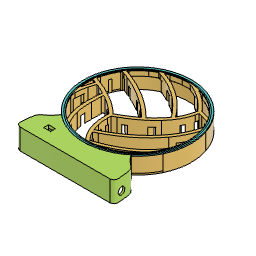
led_volleyball v4 (Autodesk Fusion 360 design; units mm, degrees)
Autodesk Fusion 360 part; units mm, degrees
(part 1 of 2)
sketch "Sketch1" plane through (0, 0, 0) normal (0, 0, 1) x (1, 0, 0) in component "volleyball"
  spline S0 degree 3 poles (6.9428, 90.0762) (-13.5515, 87.9678) (-33.2869, 78.5218) (-48.0462, 63.7625) knots 0 0 0 0 1 1 1 1
  spline S1 degree 3 poles (-48.0462, 63.7625) (-69.5526, 42.2982) (-78.872, 11.9784) (-73.137, -17.8354) knots 0 0 0 0 1 1 1 1
  spline S2 degree 3 poles (-73.137, -17.8354) (-69.7213, -35.5888) (-61.0344, -51.9084) (-48.0883, -64.8544) knots 0 0 0 0 1 1 1 1
  spline S3 degree 3 poles (-48.0883, -64.8544) (-27.594, -85.3066) (1.5451, -94.9212) (29.9252, -90.5778) knots 0 0 0 0 1 1 1 1
  spline S4 degree 3 poles (29.9252, -90.5778) (59.4438, -86.0656) (85.2093, -66.9629) (98.2397, -39.9744) knots 0 0 0 0 1 1 1 1
  spline S5 degree 3 poles (98.2397, -39.9744) (108.5291, -18.6788) (110.0472, 5.1048) (102.6253, 27.8341) knots 0 0 0 0 1 1 1 1
  spline S6 degree 3 poles (102.6253, 27.8341) (90.354, 65.4493) (54.8473, 90.9196) (15.4189, 90.4979) knots 0 0 0 0 1 1 1 1
  spline S7 degree 3 poles (15.4189, 90.4979) (12.72, 90.4558) (8.9248, 90.2449) (6.9428, 90.0762) knots 0 0 0 0 1 1 1 1
  spline S8 degree 3 poles (20.3105, 84.1725) (28.8709, 81.4737) (39.6242, 75.4434) (48.058, 68.612) knots 0 0 0 0 1 1 1 1
  spline S9 degree 3 poles (48.058, 68.612) (52.0641, 65.3649) (60.6667, 57.0997) (63.4921, 53.7683) knots 0 0 0 0 1 1 1 1
  line L0 (63.4921, 53.7683) -> (65.1789, 51.7864)
  line L1 (65.1789, 51.7864) -> (64.2933, 47.5694)
  spline S10 degree 3 poles (64.2933, 47.5694) (62.9017, 40.7801) (59.992, 33.3583) (55.9859, 26.5268) knots 0 0 0 0 1 1 1 1
  line L2 (55.9859, 26.5268) -> (54.9317, 24.7557)
  line L3 (54.9317, 24.7557) -> (52.781, 27.5811)
  spline S11 degree 3 poles (52.781, 27.5811) (45.57, 37.2379) (35.365, 47.5694) (24.9914, 55.666) knots 0 0 0 0 1 1 1 1
  spline S12 degree 3 poles (24.9914, 55.666) (13.2261, 64.8589) (-2.1236, 73.2928) (-14.7323, 77.4676) knots 0 0 0 0 1 1 1 1
  spline S13 degree 3 poles (-14.7323, 77.4676) (-18.1902, 78.6061) (-18.3167, 78.5218) (-10.6418, 81.052) knots 0 0 0 0 1 1 1 1
  spline S14 degree 3 poles (-10.6418, 81.052) (-4.2743, 83.1183) (-0.226, 84.046) (6.0994, 84.8472) knots 0 0 0 0 1 1 1 1
  spline S15 degree 3 poles (6.0994, 84.8472) (13.4369, 85.7328) (15.7141, 85.6484) (20.3105, 84.1725) knots 0 0 0 0 1 1 1 1
  spline S16 degree 3 poles (44.0519, 80.7568) (53.2027, 77.5941) (61.1728, 73.2928) (69.0163, 67.2626) knots 0 0 0 0 1 1 1 1
  spline S17 degree 3 poles (69.0163, 67.2626) (73.3597, 63.9312) (80.2334, 57.0997) (83.3961, 53.0936) knots 0 0 0 0 1 1 1 1
  line L4 (83.3961, 53.0936) -> (85.4202, 50.5213)
  line L5 (85.4202, 50.5213) -> (83.6069, 51.1538)
  spline S18 degree 3 poles (83.6069, 51.1538) (82.5948, 51.5333) (78.9683, 52.5454) (75.5104, 53.431) knots 0 0 0 0 1 1 1 1
  line L6 (75.5104, 53.431) -> (69.185, 55.0334)
  line L7 (69.185, 55.0334) -> (65.3475, 59.2925)
  spline S19 degree 3 poles (65.3475, 59.2925) (57.3353, 68.2325) (49.4496, 74.7265) (37.7265, 82.064) knots 0 0 0 0 1 1 1 1
  line L8 (37.7265, 82.064) -> (36.2506, 82.9918)
  line L9 (36.2506, 82.9918) -> (37.7265, 82.6966)
  spline S20 degree 3 poles (37.7265, 82.6966) (38.5277, 82.5701) (41.3953, 81.6845) (44.0519, 80.7568) knots 0 0 0 0 1 1 1 1
  spline S21 degree 3 poles (-20.4252, 74.094) (-7.0574, 70.1301) (10.6116, 60.5576) (23.5998, 50.2261) knots 0 0 0 0 1 1 1 1
  spline S22 degree 3 poles (23.5998, 50.2261) (29.7987, 45.3344) (43.3772, 31.6294) (47.9737, 25.6835) knots 0 0 0 0 1 1 1 1
  spline S23 degree 3 poles (47.9737, 25.6835) (49.9978, 23.0268) (51.6425, 20.6653) (51.6425, 20.3701) knots 0 0 0 0 1 1 1 1
  spline S24 degree 3 poles (51.6425, 20.3701) (51.6425, 18.852) (37.347, 3.3336) (32.5819, -0.2508) knots 0 0 0 0 1 1 1 1
  line L10 (32.5819, -0.2508) -> (31.0638, -1.4315)
  line L11 (31.0638, -1.4315) -> (26.889, 2.6168)
  spline S25 degree 3 poles (26.889, 2.6168) (16.3466, 12.9904) (0.9548, 24.5027) (-13.2985, 32.6414) knots 0 0 0 0 1 1 1 1
  spline S26 degree 3 poles (-13.2985, 32.6414) (-23.5035, 38.503) (-38.4315, 45.4188) (-49.0582, 49.214) knots 0 0 0 0 1 1 1 1
  line L12 (-49.0582, 49.214) -> (-52.9378, 50.6056)
  line L13 (-52.9378, 50.6056) -> (-51.3776, 52.5454)
  spline S27 degree 3 poles (-51.3776, 52.5454) (-46.4016, 58.7022) (-40.6243, 64.2685) (-34.3833, 68.9493) knots 0 0 0 0 1 1 1 1
  spline S28 degree 3 poles (-34.3833, 68.9493) (-30.9254, 71.5217) (-24.5578, 75.3169) (-24.0096, 75.1482) knots 0 0 0 0 1 1 1 1
  spline S29 degree 3 poles (-24.0096, 75.1482) (-23.7566, 75.0639) (-22.1119, 74.6) (-20.4252, 74.094) knots 0 0 0 0 1 1 1 1
  spline S30 degree 3 poles (75.7212, 48.202) (81.1611, 46.726) (86.6009, 44.7019) (89.2154, 43.226) knots 0 0 0 0 1 1 1 1
  spline S31 degree 3 poles (89.2154, 43.226) (90.354, 42.5934) (91.1974, 41.497) (92.5468, 39.009) knots 0 0 0 0 1 1 1 1
  line L14 (92.5468, 39.009) -> (94.318, 35.6776)
  line L15 (94.318, 35.6776) -> (92.7999, 29.8161)
  spline S32 degree 3 poles (92.7999, 29.8161) (85.0407, -0.6303) (61.1728, -29.432) (25.413, -51.4023) knots 0 0 0 0 1 1 1 1
  spline S33 degree 3 poles (25.413, -51.4023) (20.0997, -54.6494) (5.5512, -62.4929) (4.75, -62.5351) knots 0 0 0 0 1 1 1 1
  spline S34 degree 3 poles (4.75, -62.5351) (4.3705, -62.5351) (2.1355, -55.5771) (1.2499, -51.6975) knots 0 0 0 0 1 1 1 1
  spline S35 degree 3 poles (1.2499, -51.6975) (-0.0151, -46.0468) (-0.6477, -40.3118) (-0.6477, -34.4502) knots 0 0 0 0 1 1 1 1
  line L16 (-0.6477, -34.4502) -> (-0.6477, -28.4621)
  line L17 (-0.6477, -28.4621) -> (5.7621, -24.9621)
  spline S36 degree 3 poles (5.7621, -24.9621) (22.2925, -15.8956) (38.1061, -3.793) (48.2689, 7.5506) knots 0 0 0 0 1 1 1 1
  spline S37 degree 3 poles (48.2689, 7.5506) (59.1486, 19.6532) (65.7692, 31.3763) (68.7633, 43.9007) knots 0 0 0 0 1 1 1 1
  spline S38 degree 3 poles (68.7633, 43.9007) (69.3958, 46.473) (69.944, 48.8345) (70.0283, 49.1297) knots 0 0 0 0 1 1 1 1
  spline S39 degree 3 poles (70.0283, 49.1297) (70.197, 49.7622) (69.6488, 49.8466) (75.7212, 48.202) knots 0 0 0 0 1 1 1 1
  spline S40 degree 3 poles (-43.8292, 41.7079) (-24.7686, 34.0752) (-5.4128, 22.7738) (10.7381, 9.7856) knots 0 0 0 0 1 1 1 1
  spline S41 degree 3 poles (10.7381, 9.7856) (16.3466, 5.2734) (26.1299, -3.6243) (26.4673, -4.5099) knots 0 0 0 0 1 1 1 1
  spline S42 degree 3 poles (26.4673, -4.5099) (26.889, -5.6063) (12.5092, -15.3474) (2.3885, -20.8295) knots 0 0 0 0 1 1 1 1
  line L18 (2.3885, -20.8295) -> (-2.3345, -23.4018)
  line L19 (-2.3345, -23.4018) -> (-5.3285, -20.6186)
  spline S43 degree 3 poles (-5.3285, -20.6186) (-19.0757, -7.6304) (-41.3412, 5.2313) (-64.1971, 13.37) knots 0 0 0 0 1 1 1 1
  spline S44 degree 3 poles (-64.1971, 13.37) (-68.7514, 14.9724) (-68.6249, 14.7616) (-67.2754, 20.0749) knots 0 0 0 0 1 1 1 1
  spline S45 degree 3 poles (-67.2754, 20.0749) (-65.3356, 27.7919) (-60.7813, 38.6295) (-57.1969, 44.238) knots 0 0 0 0 1 1 1 1
  line L20 (-57.1969, 44.238) -> (-55.8897, 46.22)
  line L21 (-55.8897, 46.22) -> (-52.0101, 44.8284)
  spline S46 degree 3 poles (-52.0101, 44.8284) (-49.8595, 44.0272) (-46.1907, 42.6356) (-43.8292, 41.7079) knots 0 0 0 0 1 1 1 1
  spline S47 degree 3 poles (98.7879, 23.4906) (100.7699, 16.9544) (102.2458, 6.7494) (102.2458, -0.5459) knots 0 0 0 0 1 1 1 1
  spline S48 degree 3 poles (102.2458, -0.5459) (102.2458, -7.5039) (101.4868, -12.6064) (99.8843, -16.5282) knots 0 0 0 0 1 1 1 1
  spline S49 degree 3 poles (99.8843, -16.5282) (90.5649, -39.2154) (70.9139, -58.2338) (43.0399, -71.6015) knots 0 0 0 0 1 1 1 1
  spline S50 degree 3 poles (43.0399, -71.6015) (36.2506, -74.8907) (26.8046, -78.6016) (20.7322, -80.4571) knots 0 0 0 0 1 1 1 1
  line L22 (20.7322, -80.4571) -> (16.9792, -81.5957)
  line L23 (16.9792, -81.5957) -> (15.9249, -80.5836)
  spline S51 degree 3 poles (15.9249, -80.5836) (13.4369, -78.3064) (6.4368, -67.9328) (6.985, -67.4267) knots 0 0 0 0 1 1 1 1
  spline S52 degree 3 poles (6.985, -67.4267) (7.0693, -67.3424) (10.0212, -65.8243) (13.4791, -64.0953) knots 0 0 0 0 1 1 1 1
  spline S53 degree 3 poles (13.4791, -64.0953) (39.6663, -50.8541) (63.4499, -31.414) (78.7574, -10.7931) knots 0 0 0 0 1 1 1 1
  spline S54 degree 3 poles (78.7574, -10.7931) (86.5588, -0.2508) (93.0107, 12.3157) (96.4264, 23.575) knots 0 0 0 0 1 1 1 1
  spline S55 degree 3 poles (96.4264, 23.575) (96.9746, 25.3461) (97.5228, 26.6955) (97.6915, 26.5268) knots 0 0 0 0 1 1 1 1
  spline S56 degree 3 poles (97.6915, 26.5268) (97.818, 26.3582) (98.3241, 25.0087) (98.7879, 23.4906) knots 0 0 0 0 1 1 1 1
  spline S57 degree 3 poles (-66.0104, 8.5205) (-64.7453, 8.0988) (-63.6489, 7.7193) (-63.5645, 7.6771) knots 0 0 0 0 1 1 1 1
  spline S58 degree 3 poles (-63.5645, 7.6771) (-63.4802, 7.5928) (-64.1971, 5.1048) (-65.167, 2.1529) knots 0 0 0 0 1 1 1 1
  spline S59 degree 3 poles (-65.167, 2.1529) (-66.0947, -0.8411) (-67.3176, -5.2689) (-67.8658, -7.6726) knots 0 0 0 0 1 1 1 1
  spline S60 degree 3 poles (-67.8658, -7.6726) (-69.0044, -12.9016) (-69.2574, -12.5221) (-69.6369, -4.7629) knots 0 0 0 0 1 1 1 1
  spline S61 degree 3 poles (-69.6369, -4.7629) (-69.9743, 1.689) (-69.5104, 9.7012) (-68.7935, 9.4482) knots 0 0 0 0 1 1 1 1
  spline S62 degree 3 poles (-68.7935, 9.4482) (-68.5405, 9.3639) (-67.2754, 8.9422) (-66.0104, 8.5205) knots 0 0 0 0 1 1 1 1
  spline S63 degree 3 poles (-53.486, 3.6288) (-49.6064, 1.942) (-42.1424, -1.6002) (-41.6786, -1.9797) knots 0 0 0 0 1 1 1 1
  spline S64 degree 3 poles (-41.6786, -1.9797) (-41.6364, -1.9797) (-41.8894, -4.0038) (-42.2268, -6.4497) knots 0 0 0 0 1 1 1 1
  spline S65 degree 3 poles (-42.2268, -6.4497) (-43.1123, -12.9859) (-43.4497, -27.9561) (-42.8593, -34.7032) knots 0 0 0 0 1 1 1 1
  spline S66 degree 3 poles (-42.8593, -34.7032) (-41.7207, -47.7336) (-39.2749, -58.0229) (-35.1845, -66.7098) knots 0 0 0 0 1 1 1 1
  spline S67 degree 3 poles (-35.1845, -66.7098) (-34.2989, -68.6496) (-33.582, -70.3364) (-33.6664, -70.3786) knots 0 0 0 0 1 1 1 1
  spline S68 degree 3 poles (-33.6664, -70.3786) (-33.9616, -70.7159) (-41.2147, -64.5592) (-45.01, -60.7639) knots 0 0 0 0 1 1 1 1
  spline S69 degree 3 poles (-45.01, -60.7639) (-52.3475, -53.3421) (-58.715, -43.8962) (-62.9742, -34.0285) knots 0 0 0 0 1 1 1 1
  spline S70 degree 3 poles (-62.9742, -34.0285) (-64.8296, -29.7272) (-64.9561, -29.179) (-65.0826, -25.1307) knots 0 0 0 0 1 1 1 1
  spline S71 degree 3 poles (-65.0826, -25.1307) (-65.2935, -19.8596) (-64.3658, -13.1968) (-62.426, -5.8171) knots 0 0 0 0 1 1 1 1
  spline S72 degree 3 poles (-62.426, -5.8171) (-61.1187, -0.7568) (-58.9681, 5.7795) (-58.5885, 5.7795) knots 0 0 0 0 1 1 1 1
  spline S73 degree 3 poles (-58.5885, 5.7795) (-58.5042, 5.7795) (-56.227, 4.8096) (-53.486, 3.6288) knots 0 0 0 0 1 1 1 1
  spline S74 degree 3 poles (-31.8953, -7.3774) (-23.8409, -12.1847) (-15.3648, -18.468) (-8.5334, -24.6669) knots 0 0 0 0 1 1 1 1
  line L24 (-8.5334, -24.6669) -> (-6.0454, -26.9019)
  line L25 (-6.0454, -26.9019) -> (-5.9189, -34.7032)
  spline S75 degree 3 poles (-5.9189, -34.7032) (-5.7502, -43.0949) (-5.0755, -48.4083) (-3.3465, -55.1132) knots 0 0 0 0 1 1 1 1
  spline S76 degree 3 poles (-3.3465, -55.1132) (-0.479, -65.993) (3.991, -74.6377) (11.0333, -82.9029) knots 0 0 0 0 1 1 1 1
  spline S77 degree 3 poles (11.0333, -82.9029) (14.5755, -87.0355) (14.7863, -86.7825) (8.1657, -86.15) knots 0 0 0 0 1 1 1 1
  spline S78 degree 3 poles (8.1657, -86.15) (-0.9429, -85.2222) (-10.2202, -82.7764) (-18.6119, -79.1077) knots 0 0 0 0 1 1 1 1
  spline S79 degree 3 poles (-18.6119, -79.1077) (-22.9132, -77.21) (-22.9975, -77.1679) (-25.106, -74.0895) knots 0 0 0 0 1 1 1 1
  spline S80 degree 3 poles (-25.106, -74.0895) (-29.3651, -67.8906) (-32.6543, -60.2579) (-34.805, -51.4867) knots 0 0 0 0 1 1 1 1
  spline S81 degree 3 poles (-34.805, -51.4867) (-37.1243, -42.0407) (-37.5038, -38.1611) (-37.546, -24.5825) knots 0 0 0 0 1 1 1 1
  spline S82 degree 3 poles (-37.546, -24.5825) (-37.546, -17.7511) (-37.3773, -10.4558) (-37.2086, -8.4316) knots 0 0 0 0 1 1 1 1
  spline S83 degree 3 poles (-37.2086, -8.4316) (-36.7869, -4.1304) (-37.2086, -4.2147) (-31.8953, -7.3774) knots 0 0 0 0 1 1 1 1
  spline S84 degree 3 poles (91.8721, -41.3238) (82.7214, -57.8121) (68.7633, -70.969) (52.2328, -78.6016) knots 0 0 0 0 1 1 1 1
  spline S85 degree 3 poles (52.2328, -78.6016) (44.3893, -82.2282) (33.4674, -85.2644) (25.8347, -85.9813) knots 0 0 0 0 1 1 1 1
  spline S86 degree 3 poles (25.8347, -85.9813) (20.3527, -86.4452) (20.4792, -85.8548) (26.3408, -83.8728) knots 0 0 0 0 1 1 1 1
  spline S87 degree 3 poles (26.3408, -83.8728) (44.6002, -77.6317) (61.0041, -68.734) (74.5826, -57.7699) knots 0 0 0 0 1 1 1 1
  spline S88 degree 3 poles (74.5826, -57.7699) (79.7273, -53.5951) (87.2335, -46.1311) (90.6492, -41.7455) knots 0 0 0 0 1 1 1 1
  spline S89 degree 3 poles (90.6492, -41.7455) (92.0408, -39.9744) (93.2637, -38.4985) (93.3059, -38.4985) knots 0 0 0 0 1 1 1 1
  spline S90 degree 3 poles (93.3059, -38.4985) (93.3902, -38.4985) (92.7577, -39.7636) (91.8721, -41.3238) knots 0 0 0 0 1 1 1 1
extrude "Extrude1" add sketch "Sketch1" along normal blind 25 makes body 1 in component "volleyball"
sketch "Sketch2" plane through (0, 0, 0) normal (0, 0, 1) x (1, 0, 0) in component "volleyball"
  spline S0 degree 3 poles (-48.0462, 63.7625) (-69.5526, 42.2982) (-78.872, 11.9784) (-73.137, -17.8354) knots 0 0 0 0 1 1 1 1
  spline S1 degree 3 poles (98.2397, -39.9744) (108.5291, -18.6788) (110.0472, 5.1048) (102.6253, 27.8341) knots 0 0 0 0 1 1 1 1
  line L0 (-74.7957, -0.2686) -> (107.2566, -0.2686) construction
  circle A0 centre (16.2304, -0.2686) radius 85.7831
  circle A1 centre (16.2304, -0.2686) radius 80.7831
  point P0 (83.3961, 53.0936)
  dimension "d3" = -5
  constraint coincident S0 L0.start
  constraint coincident S1 L0.end
  constraint horizontal L0
  constraint midpoint L0 A0.centre
  constraint coincident A0 P0
extrude "Extrude2" cut sketch "Sketch2" along normal blind 17 bodies 1 in component "volleyball"
copy_body "CutPasteBodies1" bodies 1 removing the originals makes body 2 in component "volleyball"
sketch "Sketch1 (2)" plane through (0, 0, 25) normal (0, 0, 1) x (-1, 0, 0) in component "top"
  spline S0 degree 3 poles (69.6369, 4.7629) (69.9743, -1.689) (69.5104, -9.7012) (68.7935, -9.4482) knots 0 0 0 0 1 1 1 1
  line L0 (68.7935, -9.4482) -> (66.0104, -8.5205)
  spline S1 degree 3 poles (66.0104, -8.5205) (64.7453, -8.0988) (63.6489, -7.7193) (63.5645, -7.6771) knots 0 0 0 0 1 1 1 1
  spline S2 degree 3 poles (63.5645, -7.6771) (63.4802, -7.5928) (64.1971, -5.1048) (65.167, -2.1529) knots 0 0 0 0 1 1 1 1
  spline S3 degree 3 poles (65.167, -2.1529) (66.0947, 0.8411) (67.3176, 5.2689) (67.8658, 7.6726) knots 0 0 0 0 1 1 1 1
  spline S4 degree 3 poles (67.8658, 7.6726) (69.0044, 12.9016) (69.2574, 12.5221) (69.6369, 4.7629) knots 0 0 0 0 1 1 1 1
  spline S5 degree 3 poles (62.426, 5.8171) (61.1187, 0.7568) (58.9681, -5.7795) (58.5885, -5.7795) knots 0 0 0 0 1 1 1 1
  spline S6 degree 3 poles (58.5885, -5.7795) (58.5042, -5.7795) (56.227, -4.8096) (53.486, -3.6288) knots 0 0 0 0 1 1 1 1
  spline S7 degree 3 poles (53.486, -3.6288) (49.6064, -1.942) (42.1424, 1.6002) (41.6786, 1.9797) knots 0 0 0 0 1 1 1 1
  spline S8 degree 3 poles (41.6786, 1.9797) (41.6364, 1.9797) (41.8894, 4.0038) (42.2268, 6.4497) knots 0 0 0 0 1 1 1 1
  spline S9 degree 3 poles (42.2268, 6.4497) (43.1123, 12.9859) (43.4497, 27.9561) (42.8593, 34.7032) knots 0 0 0 0 1 1 1 1
  spline S10 degree 3 poles (42.8593, 34.7032) (41.7207, 47.7336) (39.2749, 58.0229) (35.1845, 66.7098) knots 0 0 0 0 1 1 1 1
  spline S11 degree 3 poles (35.1845, 66.7098) (34.2989, 68.6496) (33.582, 70.3364) (33.6664, 70.3786) knots 0 0 0 0 1 1 1 1
  spline S12 degree 3 poles (33.6664, 70.3786) (33.9616, 70.7159) (41.2147, 64.5592) (45.01, 60.7639) knots 0 0 0 0 1 1 1 1
  spline S13 degree 3 poles (45.01, 60.7639) (52.3475, 53.3421) (58.715, 43.8962) (62.9742, 34.0285) knots 0 0 0 0 1 1 1 1
  spline S14 degree 3 poles (62.9742, 34.0285) (64.8296, 29.7272) (64.9561, 29.179) (65.0826, 25.1307) knots 0 0 0 0 1 1 1 1
  spline S15 degree 3 poles (65.0826, 25.1307) (65.2935, 19.8596) (64.3658, 13.1968) (62.426, 5.8171) knots 0 0 0 0 1 1 1 1
  spline S16 degree 3 poles (-90.6492, 41.7455) (-92.0408, 39.9744) (-93.2637, 38.4985) (-93.3059, 38.4985) knots 0 0 0 0 1 1 1 1
  spline S17 degree 3 poles (-93.3059, 38.4985) (-93.3902, 38.4985) (-92.7577, 39.7636) (-91.8721, 41.3238) knots 0 0 0 0 1 1 1 1
  spline S18 degree 3 poles (-91.8721, 41.3238) (-82.7214, 57.8121) (-68.7633, 70.969) (-52.2328, 78.6016) knots 0 0 0 0 1 1 1 1
  spline S19 degree 3 poles (-52.2328, 78.6016) (-44.3893, 82.2282) (-33.4674, 85.2644) (-25.8347, 85.9813) knots 0 0 0 0 1 1 1 1
  spline S20 degree 3 poles (-25.8347, 85.9813) (-20.3527, 86.4452) (-20.4792, 85.8548) (-26.3408, 83.8728) knots 0 0 0 0 1 1 1 1
  spline S21 degree 3 poles (-26.3408, 83.8728) (-44.6002, 77.6317) (-61.0041, 68.734) (-74.5826, 57.7699) knots 0 0 0 0 1 1 1 1
  spline S22 degree 3 poles (-74.5826, 57.7699) (-79.7273, 53.5951) (-87.2335, 46.1311) (-90.6492, 41.7455) knots 0 0 0 0 1 1 1 1
  spline S23 degree 3 poles (37.546, 24.5825) (37.546, 17.7511) (37.3773, 10.4558) (37.2086, 8.4316) knots 0 0 0 0 1 1 1 1
  spline S24 degree 3 poles (37.2086, 8.4316) (36.7869, 4.1304) (37.2086, 4.2147) (31.8953, 7.3774) knots 0 0 0 0 1 1 1 1
  spline S25 degree 3 poles (31.8953, 7.3774) (23.8409, 12.1847) (15.3648, 18.468) (8.5334, 24.6669) knots 0 0 0 0 1 1 1 1
  line L1 (8.5334, 24.6669) -> (6.0454, 26.9019)
  line L2 (6.0454, 26.9019) -> (5.9189, 34.7032)
  spline S26 degree 3 poles (5.9189, 34.7032) (5.7502, 43.0949) (5.0755, 48.4083) (3.3465, 55.1132) knots 0 0 0 0 1 1 1 1
  spline S27 degree 3 poles (3.3465, 55.1132) (0.479, 65.993) (-3.991, 74.6377) (-11.0333, 82.9029) knots 0 0 0 0 1 1 1 1
  spline S28 degree 3 poles (-11.0333, 82.9029) (-14.5755, 87.0355) (-14.7863, 86.7825) (-8.1657, 86.15) knots 0 0 0 0 1 1 1 1
  spline S29 degree 3 poles (-8.1657, 86.15) (0.9429, 85.2222) (10.2202, 82.7764) (18.6119, 79.1077) knots 0 0 0 0 1 1 1 1
  spline S30 degree 3 poles (18.6119, 79.1077) (22.9132, 77.21) (22.9975, 77.1679) (25.106, 74.0895) knots 0 0 0 0 1 1 1 1
  spline S31 degree 3 poles (25.106, 74.0895) (29.3651, 67.8906) (32.6543, 60.2579) (34.805, 51.4867) knots 0 0 0 0 1 1 1 1
  spline S32 degree 3 poles (34.805, 51.4867) (37.1243, 42.0407) (37.5038, 38.1611) (37.546, 24.5825) knots 0 0 0 0 1 1 1 1
  spline S33 degree 3 poles (-68.7633, -43.9007) (-69.3958, -46.473) (-69.944, -48.8345) (-70.0283, -49.1297) knots 0 0 0 0 1 1 1 1
  spline S34 degree 3 poles (-70.0283, -49.1297) (-70.197, -49.7622) (-69.6488, -49.8466) (-75.7212, -48.202) knots 0 0 0 0 1 1 1 1
  spline S35 degree 3 poles (-75.7212, -48.202) (-81.1611, -46.726) (-86.6009, -44.7019) (-89.2154, -43.226) knots 0 0 0 0 1 1 1 1
  spline S36 degree 3 poles (-89.2154, -43.226) (-90.354, -42.5934) (-91.1974, -41.497) (-92.5468, -39.009) knots 0 0 0 0 1 1 1 1
  line L3 (-92.5468, -39.009) -> (-94.318, -35.6776)
  line L4 (-94.318, -35.6776) -> (-92.7999, -29.8161)
  spline S37 degree 3 poles (-92.7999, -29.8161) (-85.0407, 0.6303) (-61.1728, 29.432) (-25.413, 51.4023) knots 0 0 0 0 1 1 1 1
  spline S38 degree 3 poles (-25.413, 51.4023) (-20.0997, 54.6494) (-5.5512, 62.4929) (-4.75, 62.5351) knots 0 0 0 0 1 1 1 1
  spline S39 degree 3 poles (-4.75, 62.5351) (-4.3705, 62.5351) (-2.1355, 55.5771) (-1.2499, 51.6975) knots 0 0 0 0 1 1 1 1
  spline S40 degree 3 poles (-1.2499, 51.6975) (0.0151, 46.0468) (0.6477, 40.3118) (0.6477, 34.4502) knots 0 0 0 0 1 1 1 1
  line L5 (0.6477, 34.4502) -> (0.6477, 28.4621)
  line L6 (0.6477, 28.4621) -> (-5.7621, 24.9621)
  spline S41 degree 3 poles (-5.7621, 24.9621) (-22.2925, 15.8956) (-38.1061, 3.793) (-48.2689, -7.5506) knots 0 0 0 0 1 1 1 1
  spline S42 degree 3 poles (-48.2689, -7.5506) (-59.1486, -19.6532) (-65.7692, -31.3763) (-68.7633, -43.9007) knots 0 0 0 0 1 1 1 1
  spline S43 degree 3 poles (10.6418, -81.052) (4.2743, -83.1183) (0.226, -84.046) (-6.0994, -84.8472) knots 0 0 0 0 1 1 1 1
  spline S44 degree 3 poles (-6.0994, -84.8472) (-13.4369, -85.7328) (-15.7141, -85.6484) (-20.3105, -84.1725) knots 0 0 0 0 1 1 1 1
  spline S45 degree 3 poles (-20.3105, -84.1725) (-28.8709, -81.4737) (-39.6242, -75.4434) (-48.058, -68.612) knots 0 0 0 0 1 1 1 1
  spline S46 degree 3 poles (-48.058, -68.612) (-52.0641, -65.3649) (-60.6667, -57.0997) (-63.4921, -53.7683) knots 0 0 0 0 1 1 1 1
  line L7 (-63.4921, -53.7683) -> (-65.1789, -51.7864)
  line L8 (-65.1789, -51.7864) -> (-64.2933, -47.5694)
  spline S47 degree 3 poles (-64.2933, -47.5694) (-62.9017, -40.7801) (-59.992, -33.3583) (-55.9859, -26.5268) knots 0 0 0 0 1 1 1 1
  line L9 (-55.9859, -26.5268) -> (-54.9317, -24.7557)
  line L10 (-54.9317, -24.7557) -> (-52.781, -27.5811)
  spline S48 degree 3 poles (-52.781, -27.5811) (-45.57, -37.2379) (-35.365, -47.5694) (-24.9914, -55.666) knots 0 0 0 0 1 1 1 1
  spline S49 degree 3 poles (-24.9914, -55.666) (-13.2261, -64.8589) (2.1236, -73.2928) (14.7323, -77.4676) knots 0 0 0 0 1 1 1 1
  spline S50 degree 3 poles (14.7323, -77.4676) (18.1902, -78.6061) (18.3167, -78.5218) (10.6418, -81.052) knots 0 0 0 0 1 1 1 1
  spline S51 degree 3 poles (34.3833, -68.9493) (30.9254, -71.5217) (24.5578, -75.3169) (24.0096, -75.1482) knots 0 0 0 0 1 1 1 1
  spline S52 degree 3 poles (24.0096, -75.1482) (23.7566, -75.0639) (22.1119, -74.6) (20.4252, -74.094) knots 0 0 0 0 1 1 1 1
  spline S53 degree 3 poles (20.4252, -74.094) (7.0574, -70.1301) (-10.6116, -60.5576) (-23.5998, -50.2261) knots 0 0 0 0 1 1 1 1
  spline S54 degree 3 poles (-23.5998, -50.2261) (-29.7987, -45.3344) (-43.3772, -31.6294) (-47.9737, -25.6835) knots 0 0 0 0 1 1 1 1
  spline S55 degree 3 poles (-47.9737, -25.6835) (-49.9978, -23.0268) (-51.6425, -20.6653) (-51.6425, -20.3701) knots 0 0 0 0 1 1 1 1
  spline S56 degree 3 poles (-51.6425, -20.3701) (-51.6425, -18.852) (-37.347, -3.3336) (-32.5819, 0.2508) knots 0 0 0 0 1 1 1 1
  line L11 (-32.5819, 0.2508) -> (-31.0638, 1.4315)
  line L12 (-31.0638, 1.4315) -> (-26.889, -2.6168)
  spline S57 degree 3 poles (-26.889, -2.6168) (-16.3466, -12.9904) (-0.9548, -24.5027) (13.2985, -32.6414) knots 0 0 0 0 1 1 1 1
  spline S58 degree 3 poles (13.2985, -32.6414) (23.5035, -38.503) (38.4315, -45.4188) (49.0582, -49.214) knots 0 0 0 0 1 1 1 1
  line L13 (49.0582, -49.214) -> (52.9378, -50.6056)
  line L14 (52.9378, -50.6056) -> (51.3776, -52.5454)
  spline S59 degree 3 poles (51.3776, -52.5454) (46.4016, -58.7022) (40.6243, -64.2685) (34.3833, -68.9493) knots 0 0 0 0 1 1 1 1
  line L15 (55.8897, -46.22) -> (52.0101, -44.8284)
  spline S60 degree 3 poles (52.0101, -44.8284) (49.8595, -44.0272) (46.1907, -42.6356) (43.8292, -41.7079) knots 0 0 0 0 1 1 1 1
  spline S61 degree 3 poles (43.8292, -41.7079) (24.7686, -34.0752) (5.4128, -22.7738) (-10.7381, -9.7856) knots 0 0 0 0 1 1 1 1
  spline S62 degree 3 poles (-10.7381, -9.7856) (-16.3466, -5.2734) (-26.1299, 3.6243) (-26.4673, 4.5099) knots 0 0 0 0 1 1 1 1
  spline S63 degree 3 poles (-26.4673, 4.5099) (-26.889, 5.6063) (-12.5092, 15.3474) (-2.3885, 20.8295) knots 0 0 0 0 1 1 1 1
  line L16 (-2.3885, 20.8295) -> (2.3345, 23.4018)
  line L17 (2.3345, 23.4018) -> (5.3285, 20.6186)
  spline S64 degree 3 poles (5.3285, 20.6186) (19.0757, 7.6304) (41.3412, -5.2313) (64.1971, -13.37) knots 0 0 0 0 1 1 1 1
  spline S65 degree 3 poles (64.1971, -13.37) (68.7514, -14.9724) (68.6249, -14.7616) (67.2754, -20.0749) knots 0 0 0 0 1 1 1 1
  spline S66 degree 3 poles (67.2754, -20.0749) (65.3356, -27.7919) (60.7813, -38.6295) (57.1969, -44.238) knots 0 0 0 0 1 1 1 1
  line L18 (57.1969, -44.238) -> (55.8897, -46.22)
  line L19 (-36.2506, -82.9918) -> (-37.7265, -82.6966)
  spline S67 degree 3 poles (-37.7265, -82.6966) (-38.5277, -82.5701) (-41.3953, -81.6845) (-44.0519, -80.7568) knots 0 0 0 0 1 1 1 1
  spline S68 degree 3 poles (-44.0519, -80.7568) (-53.2027, -77.5941) (-61.1728, -73.2928) (-69.0163, -67.2626) knots 0 0 0 0 1 1 1 1
  spline S69 degree 3 poles (-69.0163, -67.2626) (-73.3597, -63.9312) (-80.2334, -57.0997) (-83.3961, -53.0936) knots 0 0 0 0 1 1 1 1
  line L20 (-83.3961, -53.0936) -> (-85.4202, -50.5213)
  line L21 (-85.4202, -50.5213) -> (-83.6069, -51.1538)
  spline S70 degree 3 poles (-83.6069, -51.1538) (-82.5948, -51.5333) (-78.9683, -52.5454) (-75.5104, -53.431) knots 0 0 0 0 1 1 1 1
  line L22 (-75.5104, -53.431) -> (-69.185, -55.0334)
  line L23 (-69.185, -55.0334) -> (-65.3475, -59.2925)
  spline S71 degree 3 poles (-65.3475, -59.2925) (-57.3353, -68.2325) (-49.4496, -74.7265) (-37.7265, -82.064) knots 0 0 0 0 1 1 1 1
  line L24 (-37.7265, -82.064) -> (-36.2506, -82.9918)
  spline S72 degree 3 poles (-96.4264, -23.575) (-96.9746, -25.3461) (-97.5228, -26.6955) (-97.6915, -26.5268) knots 0 0 0 0 1 1 1 1
  spline S73 degree 3 poles (-97.6915, -26.5268) (-97.818, -26.3582) (-98.3241, -25.0087) (-98.7879, -23.4906) knots 0 0 0 0 1 1 1 1
  spline S74 degree 3 poles (-98.7879, -23.4906) (-100.7699, -16.9544) (-102.2458, -6.7494) (-102.2458, 0.5459) knots 0 0 0 0 1 1 1 1
  spline S75 degree 3 poles (-102.2458, 0.5459) (-102.2458, 7.5039) (-101.4868, 12.6064) (-99.8843, 16.5282) knots 0 0 0 0 1 1 1 1
  spline S76 degree 3 poles (-99.8843, 16.5282) (-90.5649, 39.2154) (-70.9139, 58.2338) (-43.0399, 71.6015) knots 0 0 0 0 1 1 1 1
  spline S77 degree 3 poles (-43.0399, 71.6015) (-36.2506, 74.8907) (-26.8046, 78.6016) (-20.7322, 80.4571) knots 0 0 0 0 1 1 1 1
  line L25 (-20.7322, 80.4571) -> (-16.9792, 81.5957)
  line L26 (-16.9792, 81.5957) -> (-15.9249, 80.5836)
  spline S78 degree 3 poles (-15.9249, 80.5836) (-13.4369, 78.3064) (-6.4368, 67.9328) (-6.985, 67.4267) knots 0 0 0 0 1 1 1 1
  spline S79 degree 3 poles (-6.985, 67.4267) (-7.0693, 67.3424) (-10.0212, 65.8243) (-13.4791, 64.0953) knots 0 0 0 0 1 1 1 1
  spline S80 degree 3 poles (-13.4791, 64.0953) (-39.6663, 50.8541) (-63.4499, 31.414) (-78.7574, 10.7931) knots 0 0 0 0 1 1 1 1
  spline S81 degree 3 poles (-78.7574, 10.7931) (-86.5588, 0.2508) (-93.0107, -12.3157) (-96.4264, -23.575) knots 0 0 0 0 1 1 1 1
  spline S82 degree 3 poles (-15.4189, -90.4979) (-12.72, -90.4558) (-8.9248, -90.2449) (-6.9428, -90.0762) knots 0 0 0 0 1 1 1 1
  spline S83 degree 3 poles (-6.9428, -90.0762) (13.5515, -87.9678) (33.2869, -78.5218) (48.0462, -63.7625) knots 0 0 0 0 1 1 1 1
  spline S84 degree 3 poles (48.0462, -63.7625) (69.5526, -42.2982) (78.872, -11.9784) (73.137, 17.8354) knots 0 0 0 0 1 1 1 1
  spline S85 degree 3 poles (73.137, 17.8354) (69.7213, 35.5888) (61.0344, 51.9084) (48.0883, 64.8544) knots 0 0 0 0 1 1 1 1
  spline S86 degree 3 poles (48.0883, 64.8544) (27.594, 85.3066) (-1.5451, 94.9212) (-29.9252, 90.5778) knots 0 0 0 0 1 1 1 1
  spline S87 degree 3 poles (-29.9252, 90.5778) (-59.4438, 86.0656) (-85.2093, 66.9629) (-98.2397, 39.9744) knots 0 0 0 0 1 1 1 1
  spline S88 degree 3 poles (-98.2397, 39.9744) (-108.5291, 18.6788) (-110.0472, -5.1048) (-102.6253, -27.8341) knots 0 0 0 0 1 1 1 1
  spline S89 degree 3 poles (-102.6253, -27.8341) (-90.354, -65.4493) (-54.8473, -90.9196) (-15.4189, -90.4979) knots 0 0 0 0 1 1 1 1
sketch "Sketch2 (2)" plane through (0, 0, 17) normal (0, 0, -1) x (1, 0, 0) in component "top"
  spline S0 degree 3 poles (69.0163, -67.2626) (71.1803, -65.6028) (73.9514, -63.0966) (79.1814, -57.9288) (81.578, -55.3516) (83.1659, -53.382) knots -1.542049 -1.542049 -1.542049 -1.542049 -0.765319 -0.765319 -0.03615 -0.03615 -0.03615 -0.03615
  spline S1 degree 3 poles (44.0519, -80.7568) (48.546, -79.2035) (52.8375, -77.3472) (61.2557, -72.7987) (65.2086, -70.19) (69.0163, -67.2626) knots -2.86661 -2.86661 -2.86661 -2.86661 -1.440889 -1.440889 0 0 0 0
  spline S2 degree 3 poles (37.7265, -82.6966) (38.2952, -82.6068) (39.7793, -82.1544) (41.426, -81.6483) (42.8063, -81.1918) (44.0519, -80.7568) knots -0.528811 -0.528811 -0.528811 -0.528811 -0.395811 -0.395811 0 0 0 0
  line L0 (37.7265, -82.6966) -> (36.2506, -82.9918)
  line L1 (36.2506, -82.9918) -> (37.7265, -82.064)
  spline S3 degree 3 poles (51.5912, -72.3642) (47.1467, -75.9141) (42.4736, -79.0928) (37.7265, -82.064) knots -1.680088 -1.680088 -1.680088 -1.680088 0 0 0 0
  arc A0 (32.5947, -78.8397) -> (51.5912, -72.3642) centre (16.2304, 0.2686) ccw
  spline S4 degree 3 poles (20.3105, -84.1725) (24.0935, -82.9799) (28.2983, -81.1427) (32.5947, -78.8397) knots -3.310112 -3.310112 -3.310112 -3.310112 -1.828268 -1.828268 -1.828268 -1.828268
  spline S5 degree 3 poles (6.0994, -84.8472) (9.7659, -85.2897) (12.1689, -85.4904) (16.3159, -85.2995) (18.031, -84.9045) (20.3105, -84.1725) knots -1.429968 -1.429968 -1.429968 -1.429968 -0.718267 -0.718267 0 0 0 0
  spline S6 degree 3 poles (-10.6418, -81.052) (-7.5101, -82.0682) (-4.9064, -82.8217) (0.5777, -84.0676) (3.319, -84.495) (6.0994, -84.8472) knots -1.627542 -1.627542 -1.627542 -1.627542 -0.840792 -0.840792 0 0 0 0
  spline S7 degree 3 poles (-14.7323, -77.4676) (-15.6453, -77.7682) (-16.3241, -77.983) (-16.7785, -78.2314) (-16.8496, -78.2793) (-16.9279, -78.3531) (-16.9531, -78.382) (-16.9829, -78.4355) (-16.9916, -78.4584) (-16.9991, -78.5067) (-16.9979, -78.5305) (-16.9841, -78.5864) (-16.9683, -78.6164) (-16.9185, -78.687) (-16.8755, -78.7284) (-16.2826, -79.2026) (-14.3951, -79.8146) (-10.6418, -81.052) knots -2.249128 -2.249128 -2.249128 -2.249128 -1.665038 -1.665038 -1.524699 -1.524699 -1.452388 -1.452388 -1.404031 -1.404031 -1.356031 -1.356031 -1.29069 -1.29069 -1.185593 -1.185593 0 0 0 0
  spline S8 degree 3 poles (-10.5223, -75.9561) (-11.9314, -76.4993) (-13.3375, -77.0058) (-14.7323, -77.4676) knots -0.440767 -0.440767 -0.440767 -0.440767 0 0 0 0
  arc A1 (-17.468, -73.1503) -> (-10.5223, -75.9561) centre (16.2304, 0.2686) ccw
  spline S9 degree 3 poles (-20.4252, -74.094) (-19.4608, -73.808) (-18.4739, -73.4928) (-17.468, -73.1503) knots -5.170906 -5.170906 -5.170906 -5.170906 -4.792869 -4.792869 -4.792869 -4.792869
  spline S10 degree 3 poles (-24.0096, -75.1482) (-23.8831, -75.1061) (-23.4087, -74.969) (-21.8265, -74.5097) (-21.197, -74.3256) (-20.4252, -74.094) knots -0.411954 -0.411954 -0.411954 -0.411954 -0.24175 -0.24175 0 0 0 0
  spline S11 degree 3 poles (-34.3833, -68.9493) (-32.895, -70.0564) (-30.9927, -71.3019) (-27.4561, -73.4929) (-25.6524, -74.5166) (-24.5229, -75.0174) (-24.3147, -75.103) (-24.1265, -75.1469) (-24.0848, -75.1541) (-24.0368, -75.1535) (-24.0223, -75.1522) (-24.0096, -75.1482) knots -0.471951 -0.471951 -0.471951 -0.471951 -0.28071 -0.28071 -0.054237 -0.054237 -0.01444 -0.01444 -0.004004 -0.004004 0 0 0 0
  spline S12 degree 3 poles (-51.0592, -52.9372) (-48.6615, -55.8716) (-46.0812, -58.6704) (-40.5279, -64.0283) (-37.5253, -66.5928) (-34.3833, -68.9493) knots -2.314621 -2.314621 -2.314621 -2.314621 -1.178261 -1.178261 0 0 0 0
  arc A2 (-51.0592, -52.9372) -> (83.1659, -53.382) centre (16.2304, 0.2686) ccw
  spline S13 degree 3 poles (-48.0462, -63.7625) (-69.5526, -42.2982) (-78.872, -11.9784) (-73.137, 17.8354) knots 0 0 0 0 1 1 1 1
  spline S14 degree 3 poles (-73.137, 17.8354) (-69.7213, 35.5888) (-61.0344, 51.9084) (-48.0883, 64.8544) knots 0 0 0 0 1 1 1 1
  spline S15 degree 3 poles (-48.0883, 64.8544) (-27.594, 85.3066) (1.5451, 94.9212) (29.9252, 90.5778) knots 0 0 0 0 1 1 1 1
  spline S16 degree 3 poles (29.9252, 90.5778) (59.4438, 86.0656) (85.2093, 66.9629) (98.2397, 39.9744) knots 0 0 0 0 1 1 1 1
  spline S17 degree 3 poles (98.2397, 39.9744) (108.5291, 18.6788) (110.0472, -5.1048) (102.6253, -27.8341) knots 0 0 0 0 1 1 1 1
  spline S18 degree 3 poles (102.6253, -27.8341) (90.354, -65.4493) (54.8473, -90.9196) (15.4189, -90.4979) knots 0 0 0 0 1 1 1 1
  spline S19 degree 3 poles (6.9428, -90.0762) (-13.5515, -87.9678) (-33.2869, -78.5218) (-48.0462, -63.7625) knots 0 0 0 0 1 1 1 1
  spline S20 degree 3 poles (15.4189, -90.4979) (12.72, -90.4558) (8.9248, -90.2449) (6.9428, -90.0762) knots 0 0 0 0 1 1 1 1
sketch "Sketch4" plane through (0, 0, 25) normal (0, 0, 1) x (-1, 0, 0) in component "top"
  circle A0 centre (-16.205, 0.6226) radius 90.985
  circle A1 centre (-16.205, 0.6226) radius 85.985
  circle A2 centre (-16.205, 0.6226) radius 87.985
  point P0 (73.137, 17.8354)
  point P1 (-102.6253, -27.8341)
  point P2 (-98.2397, 39.9744)
  dimension "d6" = -5
  dimension "d7" = -3
  constraint coincident A0 P0
  constraint coincident A0 P1
  constraint coincident A0 P2
extrude "Extrude1'" add sketch "Sketch4" along normal blind 2 separate body contours A0 makes body 3 in component "top"
extrude "Extrude2'" add sketch "Sketch4" along normal blind 2 contours A2 bodies 3 in component "top"
extrude "Extrude3" cut sketch "Sketch4" along normal blind 1.5 contours A2 bodies 3 in component "top"
sketch "elect" plane through (0, 0, 27) normal (0, 0, 1) x (-1, 0, 0) in component "base"
  circle A0 centre (-16.205, 0.6226) radius 85.985
  circle A1 centre (-16.205, 0.6226) radius 90.985
  circle A2 centre (-16.205, 0.6226) radius 90.985
  line L0 (16.4858, 96.7425) -> (-28.5142, 96.7425)
  line L1 (-28.5142, 96.7425) -> (-28.5142, 114.7425)
  line L2 (-28.5142, 114.7425) -> (16.4858, 114.7425)
  line L3 (16.4858, 114.7425) -> (16.4858, 96.7425)
  line L4 (23.0632, 117.9081) -> (45.0632, 117.9081)
  line L5 (45.0632, 117.9081) -> (45.0632, 95.9081)
  line L6 (45.0632, 95.9081) -> (23.0632, 95.9081)
  line L7 (23.0632, 95.9081) -> (23.0632, 117.9081)
  line L8 (23.0632, 117.9081) -> (45.0632, 95.9081) construction
  line L9 (45.0632, 117.9081) -> (23.0632, 95.9081) construction
  line L10 (-34.7004, 100.2492) -> (-89.7004, 100.2492)
  line L11 (-89.7004, 100.2492) -> (-89.7004, 118.2492)
  line L12 (-89.7004, 118.2492) -> (-34.7004, 118.2492)
  line L13 (-34.7004, 118.2492) -> (-34.7004, 100.2492)
  line L14 (74.78, 0.6226) -> (74.78, 152.1507) construction
  line L15 (-107.1899, 0.6226) -> (-107.1899, 156.1026) construction
  line L16 (74.78, 65.0514) -> (-107.1899, 65.0514) construction
  line L17 (-16.205, 65.0514) -> (-16.205, 155.0496) construction
  point P0 (34.0632, 106.9081)
  point P1 (-107.1899, 0.6226)
  dimension "d14" = 45
  dimension "d15" = 18
  dimension "d16" = 22
  dimension "d17" = 22
  dimension "d18" = 55
  dimension "d19" = 18
  dimension "d20" = 155.48
  constraint horizontal L0
  constraint vertical L1
  constraint horizontal L2
  constraint vertical L3
  constraint horizontal L4
  constraint perpendicular L4 L5
  constraint parallel L4 L6
  constraint parallel L5 L7
  constraint coincident L8 P0
  constraint coincident L9 P0
  constraint horizontal L10
  constraint vertical L11
  constraint horizontal L12
  constraint vertical L13
  constraint vertical L14
  constraint coincident A2 L14.start
  constraint vertical L15
  constraint coincident P1 L15.start
  constraint coincident L14 L16.start
  constraint coincident L15 L16.end
  constraint perpendicular L15 L16
  constraint vertical L17
  constraint midpoint L16 L17.start
  measures "d14" distance of L0.start L0.end
  measures "d15" distance of L0.start L2.end
  measures "d16" distance of L5.end L6.end
  measures "d17" distance of L4.end L5.end
  measures "d18" distance of L10.start L10.end
  measures "d19" distance of L10.start L12.end
  measures "d20" distance of P1 L15.end
extrude "Extrude1''" add sketch "elect" against normal blind 5 separate body contours L4 L5 L6 L7 makes body 4 in component "base"
extrude "Extrude2''" add sketch "elect" against normal blind 5 separate body contours L0 L1 L2 L3 makes body 5 in component "base"
extrude "Extrude3'" add sketch "elect" against normal blind 8 separate body contours L10 L11 L12 L13 makes body 6 in component "base"
sketch "housing" plane through (0, 0, 27) normal (0, 0, 1) x (-1, 0, 0) in component "base"
  line L0 (-16.205, 65.0514) -> (-16.205, 155.0496)
  line L1 (-16.205, 123.3059) -> (59.7295, 123.3059)
  spline S0 degree 5 poles (59.7295, 123.3059) (60.245, 123.1722) (61.2236, 122.8835) (62.534, 122.386) (63.9652, 121.5939) (65.2339, 120.3838) (66.0094, 118.9426) (66.3532, 117.2496) (66.3723, 115.2742) (66.1906, 112.9915) (65.9241, 110.398) (65.6562, 107.5261) (65.4064, 104.4647) (65.1391, 101.3447) (64.7868, 98.3115) (64.2681, 95.5014) (63.508, 93.0168) (62.4573, 90.9012) (61.1129, 89.1131) (59.5053, 87.5514) (57.6848, 86.0832) (55.7086, 84.5692) (53.6269, 82.8931) (51.4742, 80.9775) (49.2741, 78.7728) (47.0405, 76.2518) (45.2327, 73.9729) (43.8661, 72.1153) (42.9503, 70.8111) (42.4913, 70.1425) knots 0 0 0 0 0 0 0.04 0.08 0.12 0.16 0.2 0.24 0.28 0.32 0.36 0.4 0.44 0.48 0.52 0.56 0.6 0.64 0.68 0.72 0.76 0.8 0.84 0.88 0.92 0.96 1 1 1 1 1 1
  circle A0 centre (-16.205, 0.6226) radius 90.985
  spline S1 degree 5 poles (42.4913, 70.1425) (42.2714, 70.3291) (41.8226, 70.706) (41.1224, 71.282) (40.1346, 72.0716) (38.8092, 73.094) (37.3925, 74.1497) (35.8841, 75.2344) (34.2838, 76.3404) (32.592, 77.4564) (30.8111, 78.569) (28.9469, 79.6634) (27.0103, 80.7253) (25.0187, 81.7415) (22.9973, 82.7013) (20.9797, 83.5978) (19.0004, 84.427) (17.09, 85.188) (15.2688, 85.883) (13.542, 86.5168) (11.8919, 87.0971) (10.2785, 87.6338) (8.6519, 88.1369) (6.963, 88.6151) (5.1737, 89.0735) (3.2694, 89.5123) (1.2638, 89.9257) (-0.8104, 90.305) (-2.9077, 90.6403) (-4.9767, 90.9232) (-6.9666, 91.1489) (-8.8354, 91.3183) (-10.5512, 91.4382) (-12.0907, 91.5183) (-13.438, 91.5688) (-14.5836, 91.5986) (-15.3354, 91.6095) (-15.8063, 91.6111) (-16.079, 91.6092) (-16.205, 91.6076) knots 0 0 0 0 0 0 0.028571 0.057143 0.085714 0.114286 0.142857 0.171429 0.2 0.228571 0.257143 0.285714 0.314286 0.342857 0.371429 0.4 0.428571 0.457143 0.485714 0.514286 0.542857 0.571429 0.6 0.628571 0.657143 0.685714 0.714286 0.742857 0.771429 0.8 0.828571 0.857143 0.885714 0.914286 0.942857 0.971429 1 1 1 1 1 1
  spline S2 degree 3 poles (48.0883, 64.8544) (27.594, 85.3066) (-1.5451, 94.9212) (-29.9252, 90.5778) knots 0 0 0 0 1 1 1 1
  line L2 (-16.205, 123.3059) -> (-92.1394, 123.3059)
  spline S3 degree 5 poles (-92.1394, 123.3059) (-92.6549, 123.1722) (-93.6335, 122.8835) (-94.9439, 122.386) (-96.3751, 121.5939) (-97.6438, 120.3838) (-98.4193, 118.9426) (-98.7631, 117.2496) (-98.7822, 115.2742) (-98.6005, 112.9915) (-98.3341, 110.398) (-98.0661, 107.5261) (-97.8163, 104.4647) (-97.549, 101.3447) (-97.1967, 98.3115) (-96.678, 95.5014) (-95.918, 93.0168) (-94.8672, 90.9012) (-93.5228, 89.1131) (-91.9152, 87.5514) (-90.0947, 86.0832) (-88.1185, 84.5692) (-86.0368, 82.8931) (-83.8841, 80.9775) (-81.684, 78.7728) (-79.4504, 76.2518) (-77.6426, 73.9729) (-76.276, 72.1153) (-75.3602, 70.8111) (-74.9012, 70.1425) knots 0 0 0 0 0 0 0.04 0.08 0.12 0.16 0.2 0.24 0.28 0.32 0.36 0.4 0.44 0.48 0.52 0.56 0.6 0.64 0.68 0.72 0.76 0.8 0.84 0.88 0.92 0.96 1 1 1 1 1 1
  line L3 (50.9393, 125.5847) -> (68.5196, 121.0271)
  line L4 (47.2666, 77.0968) -> (37.716, 63.1882)
  line L5 (-83.3492, 125.5847) -> (-100.9295, 121.0271)
  line L6 (-79.6765, 77.0968) -> (-70.1259, 63.1882)
  spline S4 degree 5 poles (-74.9012, 70.1425) (-74.6813, 70.3291) (-74.2325, 70.706) (-73.5323, 71.282) (-72.5446, 72.0716) (-71.2191, 73.094) (-69.8024, 74.1497) (-68.294, 75.2344) (-66.6938, 76.3404) (-65.0019, 77.4564) (-63.221, 78.569) (-61.3568, 79.6634) (-59.4202, 80.7253) (-57.4286, 81.7415) (-55.4072, 82.7013) (-53.3896, 83.5978) (-51.4103, 84.427) (-49.4999, 85.188) (-47.6787, 85.883) (-45.9519, 86.5168) (-44.3018, 87.0971) (-42.6884, 87.6338) (-41.0618, 88.1369) (-39.3729, 88.6151) (-37.5836, 89.0735) (-35.6793, 89.5123) (-33.6737, 89.9257) (-31.5995, 90.305) (-29.5022, 90.6403) (-27.4332, 90.9232) (-25.4433, 91.1489) (-23.5745, 91.3183) (-21.8587, 91.4382) (-20.3192, 91.5183) (-18.9719, 91.5688) (-17.8263, 91.5986) (-17.0745, 91.6095) (-16.6036, 91.6111) (-16.331, 91.6092) (-16.205, 91.6076) knots 0 0 0 0 0 0 0.028571 0.057143 0.085714 0.114286 0.142857 0.171429 0.2 0.228571 0.257143 0.285714 0.314286 0.342857 0.371429 0.4 0.428571 0.457143 0.485714 0.514286 0.542857 0.571429 0.6 0.628571 0.657143 0.685714 0.714286 0.742857 0.771429 0.8 0.828571 0.857143 0.885714 0.914286 0.942857 0.971429 1 1 1 1 1 1
  line L7 (46.9604, 66.3492) -> (38.0221, 73.9359)
  line L8 (-11.5983, 91.6605) -> (-20.8116, 91.5546)
  line L9 (-79.3703, 66.3492) -> (-70.432, 73.9359)
  line L10 (-20.8116, 91.6605) -> (-11.5983, 91.5546)
  spline S5 degree 3 poles (-74.3128, 74.4884) (-72.7312, 75.7276) (-70.9632, 77.04) (-68.9809, 78.3998) (-66.3588, 80.1985) (-63.3259, 82.0727) (-60.0803, 83.7465) (-57.1798, 85.2424) (-54.1529, 86.5606) (-51.4129, 87.6508) (-49.085, 88.5771) (-46.996, 89.345) (-44.9825, 90.0266) (-42.8385, 90.7523) (-40.7016, 91.392) (-38.2557, 91.9856) (-35.5659, 92.6384) (-32.4966, 93.2301) (-29.4974, 93.6607) (-26.5311, 94.0867) (-23.7079, 94.3344) (-21.476, 94.4585) (-19.356, 94.5764) (-17.7702, 94.6076) (-16.6832, 94.6099) (-16.5128, 94.6102) (-16.3539, 94.6095) (-16.205, 94.6078) knots 0.058463 0.058463 0.058463 0.058463 0.160675 0.160675 0.160675 0.295879 0.295879 0.295879 0.416706 0.416706 0.416706 0.519365 0.519365 0.519365 0.62868 0.62868 0.62868 0.748891 0.748891 0.748891 0.867785 0.867785 0.867785 0.980719 0.980719 0.980719 0.998422 0.998422 0.998422 0.998422
  spline S6 degree 3 poles (41.9029, 74.4884) (40.3213, 75.7276) (38.5533, 77.04) (36.571, 78.3998) (33.9489, 80.1985) (30.916, 82.0727) (27.6704, 83.7465) (24.7699, 85.2424) (21.743, 86.5606) (19.003, 87.6508) (16.6751, 88.5771) (14.5861, 89.345) (12.5726, 90.0266) (10.4286, 90.7523) (8.2917, 91.392) (5.8457, 91.9856) (3.156, 92.6384) (0.0867, 93.2301) (-2.9125, 93.6607) (-5.8788, 94.0867) (-8.702, 94.3344) (-10.9339, 94.4585) (-13.0539, 94.5764) (-14.6397, 94.6076) (-15.7267, 94.6099) (-15.8971, 94.6102) (-16.056, 94.6095) (-16.205, 94.6078) knots 0.058463 0.058463 0.058463 0.058463 0.160675 0.160675 0.160675 0.295879 0.295879 0.295879 0.416706 0.416706 0.416706 0.519365 0.519365 0.519365 0.62868 0.62868 0.62868 0.748891 0.748891 0.748891 0.867785 0.867785 0.867785 0.980719 0.980719 0.980719 0.998422 0.998422 0.998422 0.998422
  spline S7 degree 3 poles (59.3314, 120.3059) (60.6475, 119.9342) (61.5712, 119.4815) (62.1242, 119.0738) (62.6402, 118.6933) (62.8527, 118.4018) (63.0241, 118.0028) (63.1977, 117.5987) (63.3211, 116.9915) (63.3329, 116.0319) (63.353, 114.3873) (63.0404, 111.8027) (62.7706, 108.8469) (62.4268, 105.0789) (62.1801, 100.752) (61.5513, 97.4831) (61.2112, 95.7151) (60.7545, 94.2865) (60.1669, 93.1545) (59.4581, 91.789) (58.5476, 90.7623) (57.235, 89.6194) (55.4378, 88.0547) (52.9174, 86.2955) (50.2842, 83.9047) (47.5599, 81.4314) (44.7254, 78.3075) (41.9029, 74.4884) knots 0.006585 0.006585 0.006585 0.006585 0.081823 0.081823 0.081823 0.152036 0.152036 0.152036 0.223139 0.223139 0.223139 0.345002 0.345002 0.345002 0.500349 0.500349 0.500349 0.584371 0.584371 0.584371 0.685733 0.685733 0.685733 0.824507 0.824507 0.824507 0.968078 0.968078 0.968078 0.968078
  line L11 (-16.205, 120.3059) -> (59.3314, 120.3059)
  line L12 (-16.205, 120.3059) -> (-91.7413, 120.3059)
  spline S8 degree 3 poles (-91.7413, 120.3059) (-93.0574, 119.9342) (-93.9811, 119.4815) (-94.5341, 119.0738) (-95.0501, 118.6933) (-95.2626, 118.4018) (-95.434, 118.0028) (-95.6076, 117.5987) (-95.731, 116.9915) (-95.7428, 116.0319) (-95.763, 114.3873) (-95.4503, 111.8027) (-95.1805, 108.8469) (-94.8367, 105.0789) (-94.5901, 100.752) (-93.9612, 97.4831) (-93.6211, 95.7151) (-93.1644, 94.2865) (-92.5768, 93.1545) (-91.868, 91.789) (-90.9576, 90.7623) (-89.6449, 89.6194) (-87.8478, 88.0547) (-85.3273, 86.2955) (-82.6941, 83.9047) (-79.9698, 81.4314) (-77.1353, 78.3075) (-74.3128, 74.4884) knots 0.006585 0.006585 0.006585 0.006585 0.081823 0.081823 0.081823 0.152036 0.152036 0.152036 0.223139 0.223139 0.223139 0.345002 0.345002 0.345002 0.500349 0.500349 0.500349 0.584371 0.584371 0.584371 0.685733 0.685733 0.685733 0.824507 0.824507 0.824507 0.968078 0.968078 0.968078 0.968078
  point P0 (65.8479, 119.023)
  point P1 (65.8479, 109.5395)
  point P2 (63.4005, 93.0198)
  point P3 (56.3643, 85.0659)
  point P4 (36.2167, 74.9881)
  point P5 (25.6297, 81.4194)
  point P6 (14.2198, 86.2646)
  point P7 (5.8201, 88.9015)
  point P8 (-5.783, 91.0087)
  point P9 (-13.5657, 91.5693)
  point P10 (-98.2578, 119.023)
  point P11 (-98.2578, 109.5395)
  point P12 (-95.8104, 93.0198)
  point P13 (-88.7743, 85.0659)
  point P14 (-68.6266, 74.9881)
  point P15 (-58.0396, 81.4194)
  point P16 (-46.6297, 86.2646)
  point P17 (-38.23, 88.9015)
  point P18 (-26.6269, 91.0087)
  point P19 (-18.8442, 91.5693)
  dimension "d27" = -3
  constraint coincident L0 L1.start
  constraint perpendicular L0 L1
  constraint coincident S0.end A0
  constraint coincident A0 P4
  constraint coincident A0 P5
  constraint coincident P6 S2
  constraint coincident A0 P7
  constraint coincident A0 P8
  constraint coincident A0 P9
  constraint coincident L0 S1.end
  constraint coincident A0 S1.end
  constraint midpoint L1.end L3
  constraint midpoint S0.end L4
  constraint midpoint S0.end L7
  constraint midpoint S1.end L8
  constraint symmetric L0 L1.start L2.start
  constraint symmetric L0 L1.end L2.end
  constraint symmetric L0 P0 P10
  constraint symmetric L0 P1 P11
  constraint symmetric L0 P2 P12
  constraint symmetric L0 P3 P13
  constraint symmetric L0 S0.end S3.end
  constraint symmetric L0 P4 P14
  constraint symmetric L0 P5 P15
  constraint symmetric L0 P6 P16
  constraint symmetric L0 P7 P17
  constraint symmetric L0 P8 P18
  constraint symmetric L0 P9 P19
  constraint symmetric L0 S1.end S4.end
  constraint symmetric L0 L3.start L5.start
  constraint symmetric L0 L3.end L5.end
  constraint symmetric L0 L4.start L6.start
  constraint symmetric L0 L4.end L6.end
  constraint symmetric L0 L7.start L9.start
  constraint symmetric L0 L7.end L9.end
  constraint symmetric L0 L8.start L10.start
  constraint symmetric L0 L8.end L10.end
extrude "Extrude4" add sketch "housing" against normal blind 35 separate body contours L0 A0 L2 S3 S4 S5 L12 S8 | L0 L1 S0 A0 S1 S6 S7 L11 makes body 7 in component "base"
extrude "Extrude5" cut sketch "housing" against normal blind 5 contours L0 S5 L12 S8 | L0 S6 S7 L11 bodies 4 5 6 in component "base"
extrude "Extrude6" add sketch "housing" against normal blind 5 contours L0 S5 L12 S8 | L0 S6 S7 L11 bodies 4 5 6 7 in component "base"
ref_plane "WorkPlane1" through (98.2578, -109.5395, 27) normal (0.995572, 0.094004, 0) x (-0.094004, 0.995572, 0) in component "base"
sketch "Sketch3" plane through (98.2578, -109.5395, 27) normal (0.995572, 0.094004, 0) x (-0.094004, 0.995572, 0) in component "base"
  circle A0 centre (-0.2418, -21.0272) radius 6
  dimension "d34" = 12
  measures "d34" diameter of A0
extrude "Extrude7" cut sketch "Sketch3" along normal blind 10 and the other way blind 20 bodies 4 in component "base"
extrude "Extrude8" add 1 faces at (53.0337, -106.2492, 19) along direction (0, 0, -1) blind 1 on bodies 4 bodies 4 in component "base"
sketch "Sketch4 (2)" plane through (0, 0, 27) normal (0, 0, 1) x (-1, 0, 0) in component "base"
  line L0 (39.2526, 95.9081) -> (28.4315, 95.9081)
  line L1 (28.4315, 95.9081) -> (28.4315, 101.2764)
  line L2 (28.4315, 101.2764) -> (39.2526, 101.2764)
  line L3 (39.2526, 101.2764) -> (39.2526, 95.9081)
  line L4 (45.0632, 95.9081) -> (23.0632, 95.9081)
  line L5 (45.0632, 117.9081) -> (23.0632, 95.9081)
  constraint horizontal L0
  constraint vertical L1
  constraint horizontal L2
  constraint vertical L3
  constraint coincident L1.end L5
  constraint coincident L0.start L4
extrude "Extrude9" add sketch "elect" against normal blind 8 separate body contours L4 L5 L6 L7 makes body 8 in component "base"
extrude "Extrude10" add sketch "elect" against normal blind 8 separate body contours L0 L1 L2 L3 makes body 9 in component "base"